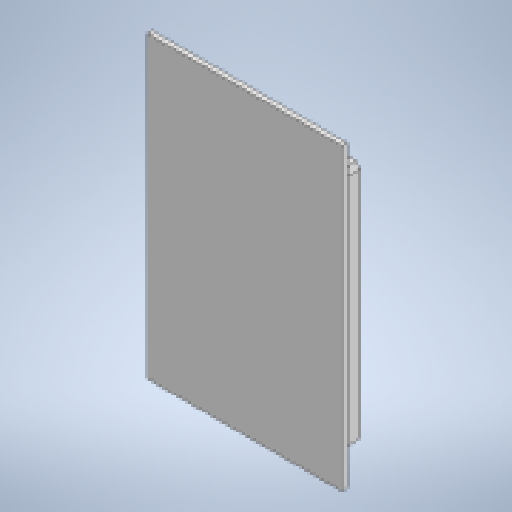
# Autodesk Inventor part: CaseButtom
Saved by Autodesk Inventor 2025.2 (Build 292293000, 293)
## iProperties
Created: 2026-02-20
Part Number: CaseButtom
Material: 一般
Document SubType Name: Modeling
Designer: naka6
Density: 1 g/cm^3
Appearance: 既定
Author: naka6
Autodesk Inventor part; units mm, degrees
ref_plane "YZ Plane" through (0, 0, 0) normal (1, 0, 0) x (0, 1, 0)
ref_plane "XZ Plane" through (0, 0, 0) normal (0, 1, 0) x (-1, 0, 0)
ref_plane "XY Plane" through (0, 0, 0) normal (0, 0, 1) x (1, 0, 0)
sketch "スケッチ2" plane through (0, 0, 0) normal (0, 0, 1) x (1, 0, 0)
  line L0 (-18.1069, 29.75) -> (19.4146, 29.75) projected
  line L1 (-19.1069, 28.75) -> (-18.1069, 29.75) projected
  line L2 (-19.1069, -20) -> (-19.1069, 28.75) projected
  line L3 (-17.5069, 29.15) -> (18.8146, 29.15) projected
  line L4 (19.8146, 28.15) -> (18.8146, 29.15) projected
  line L5 (19.8146, 28.15) -> (19.8146, -19.4) projected
  line L6 (18.8146, -20.4) -> (19.8146, -19.4) projected
  line L7 (18.8146, -20.4) -> (-17.5069, -20.4) projected
  line L8 (-18.5069, -19.4) -> (-17.5069, -20.4) projected
  line L9 (-18.5069, -19.4) -> (-18.5069, 28.15) projected
  line L10 (-17.5069, 29.15) -> (-18.5069, 28.15) projected
  line L11 (18.7318, 28.95) -> (-17.424, 28.95)
  line L12 (-17.424, 28.95) -> (-18.3069, 28.0672)
  line L13 (-18.3069, 28.0672) -> (-18.3069, -19.3172)
  line L14 (-18.3069, -19.3172) -> (-17.424, -20.2)
  line L15 (-17.424, -20.2) -> (18.7318, -20.2)
  line L16 (18.7318, -20.2) -> (19.6146, -19.3172)
  line L17 (19.6146, -19.3172) -> (19.6146, 28.0672)
  line L18 (19.6146, 28.0672) -> (18.7318, 28.95)
  line L19 (-17.1341, 28.25) -> (18.4418, 28.25)
  line L20 (18.4418, 28.25) -> (18.9146, 27.7772)
  line L21 (18.9146, 27.7772) -> (18.9146, -19.0272)
  line L22 (18.9146, -19.0272) -> (18.4418, -19.5)
  line L23 (18.4418, -19.5) -> (-17.1341, -19.5)
  line L24 (-17.1341, -19.5) -> (-17.6069, -19.0272)
  line L25 (-17.6069, -19.0272) -> (-17.6069, 27.7772)
  line L26 (-17.6069, 27.7772) -> (-17.1341, 28.25)
  line L27 (20.4146, 34.75) -> (20.4146, -26) projected
  line L28 (-19.1069, 34.75) -> (20.4146, 34.75) projected
  line L29 (-19.1069, 34.75) -> (-19.1069, -26) projected
  line L30 (20.4146, -26) -> (-19.1069, -26) projected
  point P0 (0, 0)
  point P1 (20.4146, -20)
  point P2 (20.4146, 28.75)
  dimension "d0" = 0.2
  dimension "d1" = 0.7
  constraints: 32 end point, 15 other
  measures "d0" distance between parallel lines of L3 L11
  measures "d1" distance between parallel lines of L11 L19
extrude "押し出し1" add sketch "スケッチ2" against normal blind 3.5 contours L18 L17 L16 L15 L14 L13 L12 L11
sketch "スケッチ3" plane through (0, 0, 0) normal (0, 0, 1) x (1, 0, 0)
  line L0 (-17.5069, 29.15) -> (18.8146, 29.15) projected
  line L1 (19.8146, 28.15) -> (18.8146, 29.15) projected
  line L2 (19.8146, 28.15) -> (19.8146, -19.4) projected
  line L3 (18.8146, -20.4) -> (19.8146, -19.4) projected
  line L4 (18.8146, -20.4) -> (-17.5069, -20.4) projected
  line L5 (-18.5069, -19.4) -> (-17.5069, -20.4) projected
  line L6 (-18.5069, -19.4) -> (-18.5069, 28.15) projected
  line L7 (-17.5069, 29.15) -> (-18.5069, 28.15) projected
  line L8 (20.4146, 34.75) -> (20.4146, -26) projected
  line L9 (-19.1069, 34.75) -> (20.4146, 34.75) projected
  line L10 (-19.1069, 34.75) -> (-19.1069, -26) projected
  line L11 (20.4146, -26) -> (-19.1069, -26) projected
  point P0 (0, 0)
  point P1 (-19.1069, 28.75)
  point P2 (-19.1069, -20)
  point P3 (20.4146, -20)
  point P4 (20.4146, 28.75)
extrude "押し出し2" add sketch "スケッチ3" along normal blind 1 contours L0 L1 L2 L3 L4 L5 L6 L7 | L8 L11 L10 L9
sketch "スケッチ4" plane through (20.4146, -26, 0) normal (1, 0, 0) x (0, 0, -1)
  line L0 (-1, 60.75) -> (-1, 0) projected
  line L1 (-1, 30.375) -> (0, 30.375)
  line L2 (0, 30.375) -> (92.3953, 30.375)
  circle A0 centre (460.8203, 30.375) radius 461.8203
  line L3 (-1, 0) -> (-1, 60.75) projected
  circle A1 centre (460.8203, 30.375) radius 461.9203
  line L4 (0, 0) -> (-1, 0) projected
  line L5 (0, 60.75) -> (-1, 60.75) projected
  point P0 (0, 26)
  point P1 (-0.1002, 60.75)
  point P2 (-1, 39.9861)
  point P3 (-0.1002, 0)
  point P4 (-1, 20.7639)
  dimension "d6" = 0.1
  constraints: 4 end point, 2 centre point, 2 point on line, 1 horizontal, 1 midpoint, 1 point on circle, 1 tangent
  measures "d6" radial gap between concentric circles of A0 A1
extrude "押し出し3" cut sketch "スケッチ4" against normal through all contours L5 A1 L0 | A1 L4 L0
